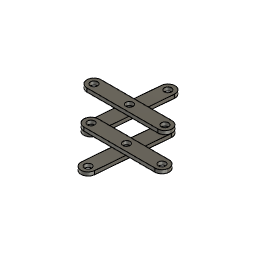
200405_jointExample_springChain_v2 (Autodesk Fusion 360 design; units mm, degrees)
Autodesk Fusion 360 part; units mm, degrees
note: some values were not read from the file. Set by a fixed rule: which sketch regions a step uses.
sketch "Sketch1" plane through (0, 0, 0) normal (0, 0, 1) x (1, 0, 0) in component "bar"
  line L0 (0, 0) -> (100, 0)
  line L1 (100, 0) -> (100, 20)
  line L2 (100, 20) -> (0, 20)
  line L3 (0, 20) -> (0, 0)
  circle A0 centre (0, 10) radius 10
  circle A1 centre (100, 10) radius 10
  circle A2 centre (0, 10) radius 5
  circle A3 centre (100, 10) radius 5
  circle A4 centre (50, 10) radius 5
  dimension "d15" = 0
  dimension "d16" = 0
  dimension "d17" = 0
  dimension "d18" = 0
  dimension "d19" = 0
  dimension "d20" = 0
  dimension "d21" = 0
  dimension "d22" = 0
  constraint horizontal L0
  constraint vertical L1
  constraint horizontal L2
  constraint vertical L3
  constraint coincident L0.start L3.end
  constraint midpoint L3 A0.centre
  constraint coincident L0.start A0
  constraint midpoint L1 A1.centre
  constraint coincident L0.end A1
  constraint concentric A0 A2
  constraint concentric A1 A3
extrude "Extrude1" add sketch "Sketch1" along normal blind 5 contours L0 L2 A0 A1 | L3 A0 A2 | L3 A0 A2 | L1 A1 A3 | L1 A1 A3 in component "bar"
component "bar" placed x (0, 1, 0) y (-1, 0, 0) z (0, 0, 1) at (60, -40, 10)
component "bar" placed x (1, 0, 0) y (0, 1, 0) z (0, 0, 1) at (0, 0, 15)
component "bar" placed x (0, -1, 0) y (1, 0, 0) z (0, 0, 1) at (-10, 110, 10)
component "bar" placed x (1, 0, 0) y (0, 1, 0) z (0, 0, 1) at (-50, 50, 15)
